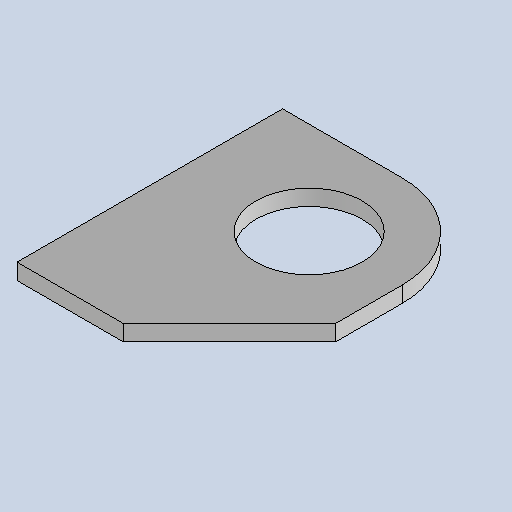
# Autodesk Inventor part: GnG frame 4.1 D-ring
Saved by Autodesk Inventor 2025.3 (Build 293356030, 356C)
## iProperties
Created: 2025-10-28
Part Number: GnG frame 4.1 D-ring
Material: Stainless Steel
Document SubType Name: Sheet Metal
Designer: admin
Stock Number: 1.4
Mass: 272.663 g
Surface Area: 140.442 cm^2
Volume: 34.0829 cm^3
Density: 8 g/cm^3
Flat Pattern Width: 8 cm
Flat Pattern Length: 10 cm
Flat Pattern Area: 80 cm^2
Sheet Metal Rule: AISI304 3mm Die 32
Sheet Metal Width: 80,000 mm
Sheet Metal Length: 100,000 mm
Sheet Metal Area: 8000,000 mm^2
Appearance: Default
Author: admin
Autodesk Inventor part; units mm, degrees
ref_plane "YZ Plane" through (0, 0, 0) normal (1, 0, 0) x (0, 1, 0)
ref_plane "XZ Plane" through (0, 0, 0) normal (0, 1, 0) x (-1, 0, 0)
ref_plane "XY Plane" through (0, 0, 0) normal (0, 0, 1) x (1, 0, 0)
sketch "Sketch6" plane through (0, 0, 0) normal (0, 0, 1) x (1, 0, 0)
  line L0 (0, 0) -> (0, 80)
  line L1 (0, 80) -> (45, 80)
  arc A0 (80, 45) -> (45, 80) centre (45, 45) ccw
  line L2 (80, 45) -> (80, 20)
  line L3 (80, 20) -> (40, -20)
  line L4 (40, -20) -> (0, -20)
  line L5 (0, -20) -> (0, 0)
  circle A1 centre (45, 45) radius 20
  dimension "d41" = 80
  dimension "d42" = 15
  dimension "d43" = 40
  dimension "d44" = 35
  dimension "d45" = 45
  dimension "d47" = 20
  dimension "d48" = 135
  dimension "d49" = 40
  measures "d41" distance of L0.start L0.end
  measures "d42" radial gap between concentric circles of A0 A1
  measures "d43" diameter of A1
  measures "d44" distance from line of L1 A0.centre
  measures "d45" distance from line of L0 A0.centre
  measures "d47" distance from line of L0.start L4
  measures "d48" angle of L4 L3
  measures "d49" distance of L3.end L4.end
extrude "Plate3" add sketch "Sketch6" along normal mid plane 6
equation "\"d46\" = Thickness"
equation "\"BendReliefWidth\" = Thickness"
equation "\"BendReliefDepth\" = 0.5 * Thickness"
equation "\"CornerReliefSize\" = 4 * Thickness"
equation "\"MinimumRemnant\" = 2 * Thickness"
equation "\"TransitionRadius\" = BendRadius"
equation "\"JacobiRadiusSize\" = BendRadius"
equation "\"GapSize\" = Thickness"
equation "\"Thickness\" = 6"
equation "\"BendRadius\" = 5"
body "Solid2"
